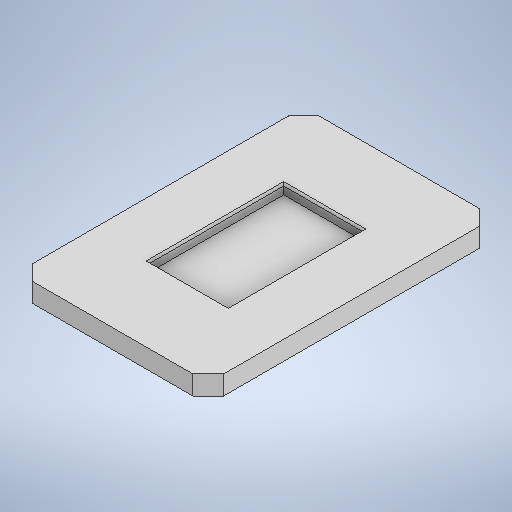
# Autodesk Inventor part: pallet
Saved by Autodesk Inventor 2025 (Build 290162000, 162)
## iProperties
Created: 2024-09-26
Part Number: pallet
Material: Generic
Document SubType Name: Modeling
Designer: DMIADX
Density: 1 g/cm^3
Appearance: Default
Author: DMIADX
Autodesk Inventor part; units mm, degrees
ref_plane "YZ Plane" through (0, 0, 0) normal (1, 0, 0) x (0, 1, 0)
ref_plane "XZ Plane" through (0, 0, 0) normal (0, 1, 0) x (-1, 0, 0)
ref_plane "XY Plane" through (0, 0, 0) normal (0, 0, 1) x (1, 0, 0)
sketch "Sketch1" plane through (0, 0, 0) normal (0, 1, 0) x (-1, 0, 0)
  line L0 (-20.5, 35) -> (20.5, 35)
  line L1 (20.5, 35) -> (20.5, -35)
  line L2 (20.5, -35) -> (-20.5, -35)
  line L3 (-20.5, -35) -> (-20.5, 35)
  line L4 (-20.5, 35) -> (20.5, -35) construction
  line L5 (20.5, 35) -> (-20.5, -35) construction
  line L6 (-50, 75) -> (50, 75)
  line L7 (50, 75) -> (50, -75)
  line L8 (50, -75) -> (-50, -75)
  line L9 (-50, -75) -> (-50, 75)
  line L10 (-50, 75) -> (50, -75) construction
  line L11 (50, 75) -> (-50, -75) construction
  point P0 (0, 0)
  dimension "d0" = 41
  dimension "d1" = 70
  dimension "d2" = 150
  dimension "d3" = 100
  constraints: 24 end point, 4 midpoint, 4 parallel, 2 horizontal, 2 perpendicular
  measures "d0" distance of L1.end L2.end
  measures "d1" distance of L0.end L1.end
  measures "d2" distance between parallel lines of L6 L8
  measures "d3" distance between parallel lines of L9 L7
extrude "Extrusion1" add sketch "Sketch1" along normal blind 10
extrude "Extrusion2" add sketch "Sketch1" along normal blind 5 contours L0 L1 L2 L3
chamfer "Chamfer1" distance 1 angle 45 4 edges at (-20.5, 10, 0) (0, 10, 35) (0, 10, -35) (20.5, 10, 0)
chamfer "Chamfer2" distance 8 angle 45 4 edges at (-50, 5, 75) (-50, 5, -75) (50, 5, -75) (50, 5, 75)
body "Solid1"
